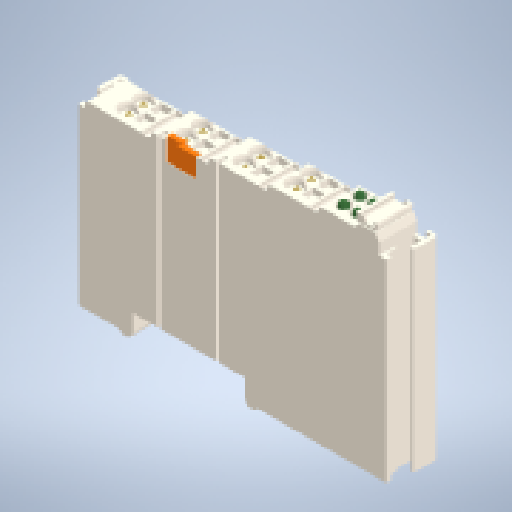
# Autodesk Inventor part: 750-408
Saved by Autodesk Inventor 2025.3 (Build 293356000, 356)
## iProperties
Category: PARTsolutions
Company: WAGO
Created: 2026-07-30
Part Number: 750-408
Material: Generic
Catalog Web Link: www.3dfindit.com
Description: 750-408-4-CHANNEL DIGITAL INPUT MODULE DC 24 V 3,0 ms
Vendor: WAGO
Document SubType Name: Modeling
Designer: psAdmin
Manufacturer: WAGO
Mass: 46.5 g
Surface Area: 195.349 cm^2
Volume: 66.2406 cm^3
Density: 1 g/cm^3
Appearance: PSOLRGB-222-214-201
Categories: <MemberInstance><Categories><Category DisplayName="" Mnemonic="CABLEANDHARNESS" InternalName="e4a7e005-5e42-4d16-b293-125e7f0d0512"><Category DisplayName="" Mnemonic="CONNECTORS" InternalName="6f634eba-a678-4820-a31d-2c2d5ee6728e"><CategoryParameter DisplayName="" Mnemonic="REFDES" InternalName="c3740e8c-60ab-4d5d-8584-52b73222f2f0"/><Category DisplayName="" Mnemonic="DISCRETEWIRE" InternalName="9a3407de-09b2-4cdb-8c40-9708d5144a28"/></Category></Category></Categories><FamilyTemplate><FamilyTemplateParameters></FamilyTemplateParameters></FamilyTemplate><CategoryParameterMap><ParamToTemplateMap><ParamToTemplate CategoryParameter="//CategoryParameter[@InternalName='c3740e8c-60ab-4d5d-8584-52b73222f2f0']" ConstantValue=""/></ParamToTemplateMap></CategoryParameterMap></MemberInstance>
PSOL_IDENT_0: {$CADENAS_DATA/23d-libs/wago/pg15/serie750/0750-0408_0999-0962.prj},156 {VTYP=3D},{NB=750-408},{LINA=
PSOL_IDENT_1: 750-408},{NN=750-408},{DATE=29.04.2026 11:59:08},{GEOMDATE=18.07.2023 08:27:45},{VERSION=},{LINEID=6
PSOL_IDENT_2: 40},{WBVAR=},{WBNUMERIC=}  {NB=750-408},{LINA=750-408},{KT=DUMMY},{BESTNR=750-408},{INFODE=Info DE},
PSOL_IDENT_3: {INFOEN=Info EN},{QUERSCHNITT1=0.08 - 2.5},{QUERSCHNITT2=28 - 14},{ABISOLIERLAENGE=8 - 9},{HOEHE=64.
PSOL_IDENT_4: 00},{BREITE=12.00},{TIEFE=100.00},{FARBE=lichtgrau},{GEWICHT=46.500},{BEMERKUNGEN=24V DC 3.0 ms  |
PSOL_IDENT_5: negativ schaltend},{RGB=0.87,0.84,0.79,0},{ECLASS71=27-24-26-04},{LINKDE=http://www.wago.com/de/p/75
PSOL_IDENT_6: 0-408},{LINKEN=http://www.wago.com/global/p/750-408},{FILENAME=750-408}
NB: 750-408
NN: 750-408
NT: 4-CHANNEL DIGITAL INPUT MODULE DC 24 V 3,0 ms
NBSYN: $BESTNR.
LINA: 750-408
CATALOG: WAGO
OFFICIAL_STANDARD_NUMBERS: NO
BESTNR: 750-408
INFODE: Info DE
INFOEN: Info EN
QUERSCHNITT1: 0.08 - 2.5
QUERSCHNITT2: 28 - 14
ABISOLIERLAENGE: 8 - 9
HOEHE: 64
BREITE: 12
TIEFE: 100
FARBE: lichtgrau
GEWICHT: 46.5
BEMERKUNGEN: 24V DC 3.0 ms  |  negativ schaltend
ECLASS71: 27-24-26-04
SUPPLIER: WAGO
ARTICLENO: 750-408
BOMINFO: 750-408
CREATOR: CADENAS GmbH
Title: 750-408
Author: Cadenas PARTsolutions
Comments: 4-CHANNEL DIGITAL INPUT MODULE DC 24 V 3,0 ms
Autodesk Inventor part; units mm, degrees
sketch "Skizze_1" plane through (0, 0, 0) normal (0, 0, 1) x (1, 0, 0)
  line L0 (-32.4, 49.7072) -> (-32.4, -6.4)
  line L1 (-32.4, -6.4) -> (-21.9679, -6.4)
  line L2 (-21.9679, -6.4) -> (-20.7, -7.1321)
  arc A0 (-20.7, -7.1321) -> (-17.7, -5.4) centre (-19.7, -5.4) ccw
  line L3 (-17.7, -5.4) -> (-17.7, 0)
  line L4 (-17.7, 0) -> (17.7, 0)
  line L5 (17.7, 0) -> (17.7, -5.4)
  arc A1 (17.7, -5.4) -> (20.7, -7.1321) centre (19.7, -5.4) ccw
  line L6 (20.7, -7.1321) -> (21.9679, -6.4)
  line L7 (21.9679, -6.4) -> (60, -6.4)
  line L8 (60, -6.4) -> (60, 57.9215)
  line L9 (60, 57.9215) -> (58.8, 60)
  line L10 (58.8, 60) -> (54.2, 60)
  arc A2 (54.2, 60) -> (53.5405, 59.7517) centre (54.2, 59) ccw
  line L11 (53.5405, 59.7517) -> (52, 58.4)
  line L12 (52, 58.4) -> (41.9117, 58.4)
  line L13 (41.9117, 58.4) -> (41.8025, 58.3537)
  line L14 (41.8025, 58.3537) -> (41.6531, 58.1989)
  arc A3 (41.6531, 58.1989) -> (41.8439, 57.6405) centre (41.8915, 57.9686) ccw
  arc A4 (42.2357, 56.9584) -> (41.8439, 57.6405) centre (41.7721, 57.1457) ccw
  line L15 (42.2357, 56.9584) -> (42.1581, 56.7664)
  line L16 (42.1581, 56.7664) -> (38.0948, 55.0416)
  line L17 (38.0948, 55.0416) -> (37.9028, 55.1192)
  arc A5 (37.6842, 55.8749) -> (37.9028, 55.1192) centre (38.0901, 55.5828) ccw
  arc A6 (37.6842, 55.8749) -> (37.4152, 56.4) centre (37.4152, 56.0685) ccw
  line L18 (37.4152, 56.4) -> (25.9117, 56.4)
  line L19 (25.9117, 56.4) -> (25.8025, 56.3537)
  line L20 (25.8025, 56.3537) -> (25.6531, 56.1989)
  arc A7 (25.6531, 56.1989) -> (25.8439, 55.6405) centre (25.8915, 55.9686) ccw
  arc A8 (26.2357, 54.9584) -> (25.8439, 55.6405) centre (25.7721, 55.1457) ccw
  line L21 (26.2357, 54.9584) -> (26.1581, 54.7664)
  line L22 (26.1581, 54.7664) -> (22.0948, 53.0416)
  line L23 (22.0948, 53.0416) -> (21.9028, 53.1192)
  arc A9 (21.6842, 53.8749) -> (21.9028, 53.1192) centre (22.0901, 53.5828) ccw
  arc A10 (21.6842, 53.8749) -> (21.4152, 54.4) centre (21.4152, 54.0685) ccw
  line L24 (21.4152, 54.4) -> (7.5117, 54.4)
  line L25 (7.5117, 54.4) -> (7.4025, 54.3537)
  line L26 (7.4025, 54.3537) -> (7.2531, 54.1989)
  arc A11 (7.2531, 54.1989) -> (7.4439, 53.6405) centre (7.4915, 53.9686) ccw
  arc A12 (7.8357, 52.9584) -> (7.4439, 53.6405) centre (7.3721, 53.1457) ccw
  line L27 (7.8357, 52.9584) -> (7.7581, 52.7664)
  line L28 (7.7581, 52.7664) -> (3.6948, 51.0416)
  line L29 (3.6948, 51.0416) -> (3.5028, 51.1192)
  arc A13 (3.2842, 51.8749) -> (3.5028, 51.1192) centre (3.6901, 51.5828) ccw
  arc A14 (3.2842, 51.8749) -> (3.0152, 52.4) centre (3.0152, 52.0685) ccw
  line L30 (3.0152, 52.4) -> (-10.8883, 52.4)
  line L31 (-10.8883, 52.4) -> (-10.9975, 52.3537)
  line L32 (-10.9975, 52.3537) -> (-11.1469, 52.1989)
  arc A15 (-11.1469, 52.1989) -> (-10.9561, 51.6405) centre (-10.9085, 51.9686) ccw
  arc A16 (-10.5643, 50.9584) -> (-10.9561, 51.6405) centre (-11.0279, 51.1457) ccw
  line L33 (-10.5643, 50.9584) -> (-10.6419, 50.7664)
  line L34 (-10.6419, 50.7664) -> (-14.7052, 49.0416)
  line L35 (-14.7052, 49.0416) -> (-14.8972, 49.1192)
  arc A17 (-15.1158, 49.8749) -> (-14.8972, 49.1192) centre (-14.7099, 49.5828) ccw
  arc A18 (-15.1158, 49.8749) -> (-15.3848, 50.4) centre (-15.3848, 50.0685) ccw
  line L36 (-15.3848, 50.4) -> (-32, 50.4)
  line L37 (-32, 50.4) -> (-32.4, 49.7072)
  constraints: 76 end point, 38 point on circle, 19 centre point
extrude "Extrusion1" add sketch "Skizze_1" along normal blind 12
sketch "Skizze_10" plane through (0, 0, 0) normal (0, 0, 1) x (1, 0, 0)
  line L0 (37.2, 56.4) -> (37.9815, 54.559)
  line L1 (37.9815, 54.559) -> (42.6932, 56.559)
  line L2 (42.6932, 56.559) -> (41.9117, 58.4)
  line L3 (41.9117, 58.4) -> (41.3423, 58.1583)
  arc A0 (41.3423, 58.1583) -> (40.8125, 56.8471) centre (41.733, 57.2378) ccw
  line L4 (40.8125, 56.8471) -> (38.9715, 56.0656)
  arc A1 (38.9715, 56.0656) -> (37.6603, 56.5954) centre (38.051, 55.6749) ccw
  line L5 (37.6603, 56.5954) -> (37.2, 56.4)
  constraints: 12 end point, 4 point on circle, 2 centre point
extrude "Extrusion2" add sketch "Skizze_10" along normal blind 0.5
sketch "Skizze_11" plane through (0, 0, 0) normal (0, 0, 1) x (1, 0, 0)
  line L0 (21.2, 54.4) -> (21.9815, 52.559)
  line L1 (21.9815, 52.559) -> (26.6932, 54.559)
  line L2 (26.6932, 54.559) -> (25.9117, 56.4)
  line L3 (25.9117, 56.4) -> (25.3423, 56.1583)
  arc A0 (25.3423, 56.1583) -> (24.8125, 54.8471) centre (25.733, 55.2378) ccw
  line L4 (24.8125, 54.8471) -> (22.9715, 54.0656)
  arc A1 (22.9715, 54.0656) -> (21.6603, 54.5954) centre (22.051, 53.6749) ccw
  line L5 (21.6603, 54.5954) -> (21.2, 54.4)
  constraints: 12 end point, 4 point on circle, 2 centre point
extrude "Extrusion3" add sketch "Skizze_11" along normal blind 0.5
sketch "Skizze_12" plane through (0, 0, 0) normal (0, 0, 1) x (1, 0, 0)
  line L0 (2.8, 52.4) -> (3.5815, 50.559)
  line L1 (3.5815, 50.559) -> (8.2932, 52.559)
  line L2 (8.2932, 52.559) -> (7.5117, 54.4)
  line L3 (7.5117, 54.4) -> (6.9423, 54.1583)
  arc A0 (6.9423, 54.1583) -> (6.4125, 52.8471) centre (7.333, 53.2378) ccw
  line L4 (6.4125, 52.8471) -> (4.5715, 52.0656)
  arc A1 (4.5715, 52.0656) -> (3.2603, 52.5954) centre (3.651, 51.6749) ccw
  line L5 (3.2603, 52.5954) -> (2.8, 52.4)
  constraints: 12 end point, 4 point on circle, 2 centre point
extrude "Extrusion4" add sketch "Skizze_12" along normal blind 0.5
sketch "Skizze_13" plane through (0, 0, 0) normal (0, 0, 1) x (1, 0, 0)
  line L0 (-15.6, 50.4) -> (-14.8185, 48.559)
  line L1 (-14.8185, 48.559) -> (-10.1068, 50.559)
  line L2 (-10.1068, 50.559) -> (-10.8883, 52.4)
  line L3 (-10.8883, 52.4) -> (-11.4577, 52.1583)
  arc A0 (-11.4577, 52.1583) -> (-11.9875, 50.8471) centre (-11.067, 51.2378) ccw
  line L4 (-11.9875, 50.8471) -> (-13.8285, 50.0656)
  arc A1 (-13.8285, 50.0656) -> (-15.1397, 50.5954) centre (-14.749, 49.6749) ccw
  line L5 (-15.1397, 50.5954) -> (-15.6, 50.4)
  constraints: 12 end point, 4 point on circle, 2 centre point
extrude "Extrusion5" add sketch "Skizze_13" along normal blind 0.5
sketch "Skizze_14" plane through (0, 0, 12) normal (0, 0, 1) x (1, 0, 0)
  line L0 (37.2, 56.4) -> (37.9815, 54.559)
  line L1 (37.9815, 54.559) -> (42.6932, 56.559)
  line L2 (42.6932, 56.559) -> (41.9117, 58.4)
  line L3 (41.9117, 58.4) -> (41.3423, 58.1583)
  arc A0 (41.3423, 58.1583) -> (40.8125, 56.8471) centre (41.733, 57.2378) ccw
  line L4 (40.8125, 56.8471) -> (38.9715, 56.0656)
  arc A1 (38.9715, 56.0656) -> (37.6603, 56.5954) centre (38.051, 55.6749) ccw
  line L5 (37.6603, 56.5954) -> (37.2, 56.4)
  constraints: 12 end point, 4 point on circle, 2 centre point
extrude "Extrusion6" add sketch "Skizze_14" against normal blind 0.5
sketch "Skizze_15" plane through (0, 0, 12) normal (0, 0, 1) x (1, 0, 0)
  line L0 (21.2, 54.4) -> (21.9815, 52.559)
  line L1 (21.9815, 52.559) -> (26.6932, 54.559)
  line L2 (26.6932, 54.559) -> (25.9117, 56.4)
  line L3 (25.9117, 56.4) -> (25.3423, 56.1583)
  arc A0 (25.3423, 56.1583) -> (24.8125, 54.8471) centre (25.733, 55.2378) ccw
  line L4 (24.8125, 54.8471) -> (22.9715, 54.0656)
  arc A1 (22.9715, 54.0656) -> (21.6603, 54.5954) centre (22.051, 53.6749) ccw
  line L5 (21.6603, 54.5954) -> (21.2, 54.4)
  constraints: 12 end point, 4 point on circle, 2 centre point
extrude "Extrusion7" add sketch "Skizze_15" against normal blind 0.5
sketch "Skizze_16" plane through (0, 0, 12) normal (0, 0, 1) x (1, 0, 0)
  line L0 (2.8, 52.4) -> (3.5815, 50.559)
  line L1 (3.5815, 50.559) -> (8.2932, 52.559)
  line L2 (8.2932, 52.559) -> (7.5117, 54.4)
  line L3 (7.5117, 54.4) -> (6.9423, 54.1583)
  arc A0 (6.9423, 54.1583) -> (6.4125, 52.8471) centre (7.333, 53.2378) ccw
  line L4 (6.4125, 52.8471) -> (4.5715, 52.0656)
  arc A1 (4.5715, 52.0656) -> (3.2603, 52.5954) centre (3.651, 51.6749) ccw
  line L5 (3.2603, 52.5954) -> (2.8, 52.4)
  constraints: 12 end point, 4 point on circle, 2 centre point
extrude "Extrusion8" add sketch "Skizze_16" against normal blind 0.5
sketch "Skizze_17" plane through (0, 0, 12) normal (0, 0, 1) x (1, 0, 0)
  line L0 (-15.6, 50.4) -> (-14.8185, 48.559)
  line L1 (-14.8185, 48.559) -> (-10.1068, 50.559)
  line L2 (-10.1068, 50.559) -> (-10.8883, 52.4)
  line L3 (-10.8883, 52.4) -> (-11.4577, 52.1583)
  arc A0 (-11.4577, 52.1583) -> (-11.9875, 50.8471) centre (-11.067, 51.2378) ccw
  line L4 (-11.9875, 50.8471) -> (-13.8285, 50.0656)
  arc A1 (-13.8285, 50.0656) -> (-15.1397, 50.5954) centre (-14.749, 49.6749) ccw
  line L5 (-15.1397, 50.5954) -> (-15.6, 50.4)
  constraints: 12 end point, 4 point on circle, 2 centre point
extrude "Extrusion9" add sketch "Skizze_17" against normal blind 0.5
sketch "Skizze_46" plane through (0, 0, 12) normal (0, 0, 1) x (1, 0, 0)
  line L0 (-7.3, 46.4) -> (2.5, 46.4)
  line L1 (2.5, 46.4) -> (2.5, 52.4)
  line L2 (2.5, 52.4) -> (-7.3, 52.4)
  line L3 (-7.3, 52.4) -> (-7.3, 46.4)
  constraints: 8 end point
extrude "Extrusion10" cut sketch "Skizze_46" against normal blind 1.9
sketch "Skizze_47" plane through (0, 0, 11.05) normal (0, 0, 1) x (1, 0, 0)
  line L0 (-7, 53.4) -> (-7, 46.6)
  arc A0 (-7, 46.6) -> (-6.8, 46.4) centre (-6.8, 46.6) ccw
  line L1 (-6.8, 46.4) -> (2, 46.4)
  arc A1 (2, 46.4) -> (2.2, 46.6) centre (2, 46.6) ccw
  line L2 (2.2, 46.6) -> (2.2, 52.2)
  arc A2 (2.2, 52.2) -> (2, 52.4) centre (2, 52.2) ccw
  line L3 (2, 52.4) -> (-3.3, 52.4)
  arc A3 (-3.3305, 52.9984) -> (-3.3, 52.4) centre (-3.3, 52.7) ccw
  line L4 (-3.3305, 52.9984) -> (-2.3246, 53.1013)
  arc A4 (-2.3246, 53.1013) -> (-2.35, 53.6) centre (-2.35, 53.35) ccw
  line L5 (-2.35, 53.6) -> (-6.8, 53.6)
  arc A5 (-6.8, 53.6) -> (-7, 53.4) centre (-6.8, 53.4) ccw
  constraints: 12 end point, 12 point on circle, 6 centre point
extrude "Extrusion11" add sketch "Skizze_47" along normal mid plane 1.6
sketch "Skizze_2" plane through (0, -6.4, 0) normal (0, 1, 0) x (1, 0, 0)
  line L0 (60, 0) -> (60, -1.7)
  arc A0 (60.5, -1.2) -> (60, -1.7) centre (60.5, -1.7) ccw
  line L1 (60.5, -1.2) -> (61.9, -1.2)
  arc A1 (62.4, -1.7) -> (61.9, -1.2) centre (61.9, -1.7) ccw
  line L2 (62.4, -1.7) -> (62.4, -4.3)
  arc A2 (62.4, -4.3) -> (63.8, -4.3) centre (63.1, -4.3) ccw
  line L3 (63.8, -4.3) -> (63.8, 1.8)
  arc A3 (63.8, 1.8) -> (62.8, 2.8) centre (62.8, 1.8) ccw
  line L4 (62.8, 2.8) -> (61.3, 2.8)
  arc A4 (61.3, 2.8) -> (60.8, 2.3) centre (61.3, 2.3) ccw
  line L5 (60.8, 2.3) -> (60.8, 1.9)
  arc A5 (60.8, 1.9) -> (61, 1.7) centre (61, 1.9) ccw
  line L6 (61, 1.7) -> (62.2, 1.7)
  arc A6 (62.4, 1.5) -> (62.2, 1.7) centre (62.2, 1.5) ccw
  line L7 (62.4, 1.5) -> (62.4, 0.2)
  arc A7 (62.2, 0) -> (62.4, 0.2) centre (62.2, 0.2) ccw
  line L8 (62.2, 0) -> (60, 0)
  constraints: 18 end point, 16 point on circle, 8 centre point
extrude "Extrusion12" add sketch "Skizze_2" along normal blind 60.8
sketch "Skizze_3" plane through (0, -6.4, 0) normal (0, 1, 0) x (1, 0, 0)
  arc A0 (-36.2, -4.3) -> (-34.8, -4.3) centre (-35.5, -4.3) ccw
  line L0 (-34.8, -4.3) -> (-34.8, -1.7)
  arc A1 (-34.3, -1.2) -> (-34.8, -1.7) centre (-34.3, -1.7) ccw
  line L1 (-34.3, -1.2) -> (-32.9, -1.2)
  arc A2 (-32.4, -1.7) -> (-32.9, -1.2) centre (-32.9, -1.7) ccw
  line L2 (-32.4, -1.7) -> (-32.4, 0)
  line L3 (-32.4, 0) -> (-34.6, 0)
  arc A3 (-34.8, 0.2) -> (-34.6, 0) centre (-34.6, 0.2) ccw
  line L4 (-34.8, 0.2) -> (-34.8, 1.5)
  arc A4 (-34.6, 1.7) -> (-34.8, 1.5) centre (-34.6, 1.5) ccw
  line L5 (-34.6, 1.7) -> (-33.4, 1.7)
  arc A5 (-33.4, 1.7) -> (-33.2, 1.9) centre (-33.4, 1.9) ccw
  line L6 (-33.2, 1.9) -> (-33.2, 2.3)
  arc A6 (-33.2, 2.3) -> (-33.7, 2.8) centre (-33.7, 2.3) ccw
  line L7 (-33.7, 2.8) -> (-35.2, 2.8)
  arc A7 (-35.2, 2.8) -> (-36.2, 1.8) centre (-35.2, 1.8) ccw
  line L8 (-36.2, 1.8) -> (-36.2, -4.3)
  constraints: 18 end point, 16 point on circle, 8 centre point
extrude "Extrusion13" add sketch "Skizze_3" along normal blind 54.8
sketch "Skizze_9" plane through (0, -6.4, 0) normal (0, 1, 0) x (1, 0, 0)
  line L0 (-34.6, -10.6) -> (-34.6, -11.8)
  arc A0 (-34.6, -11.8) -> (-34.4, -12) centre (-34.4, -11.8) ccw
  line L1 (-34.4, -12) -> (-32.4, -12)
  line L2 (-32.4, -12) -> (-32.4, -7)
  line L3 (-32.4, -7) -> (-33, -7)
  line L4 (-33, -7) -> (-33, -10.4)
  line L5 (-33, -10.4) -> (-34.4, -10.4)
  arc A1 (-34.4, -10.4) -> (-34.6, -10.6) centre (-34.4, -10.6) ccw
  constraints: 12 end point, 4 point on circle, 2 centre point
extrude "Extrusion14" add sketch "Skizze_9" along normal blind 54.8
sketch "Skizze_8" plane through (0, -6.4, 0) normal (0, 1, 0) x (1, 0, 0)
  line L0 (60, -7) -> (60, -12)
  line L1 (60, -12) -> (62, -12)
  arc A0 (62, -12) -> (62.2, -11.8) centre (62, -11.8) ccw
  line L2 (62.2, -11.8) -> (62.2, -10.6)
  arc A1 (62.2, -10.6) -> (62, -10.4) centre (62, -10.6) ccw
  line L3 (62, -10.4) -> (60.6, -10.4)
  line L4 (60.6, -10.4) -> (60.6, -7)
  line L5 (60.6, -7) -> (60, -7)
  constraints: 12 end point, 4 point on circle, 2 centre point
extrude "Extrusion15" add sketch "Skizze_8" along normal blind 60.8
sketch "Skizze_4" plane through (49, 0, 0) normal (1, 0, 0) x (0, 0, -1)
  line L0 (-2.7, 56.4) -> (-2.7, 58.4)
  line L1 (-2.7, 58.4) -> (-0.6, 58.4)
  line L2 (-0.6, 58.4) -> (-0.6, 58)
  line L3 (-0.6, 58) -> (-1, 57.6)
  line L4 (-1, 57.6) -> (-1, 56.4)
  line L5 (-1, 56.4) -> (-2.7, 56.4)
  line L6 (-2.7, 56.4) -> (-2.7, 58.4)
  constraints: 14 end point
revolve "Revolution1" cut sketch "Skizze_4" angle 360 about axis through (49, 56.4, 2.7) along (0, -1, 0)
pattern_linear "Rectangular Pattern1" count 2 spacing 5 along (0, 0, 1) of "Revolution1"
sketch "Skizze_6" plane through (49, 0, 0) normal (1, 0, 0) x (0, 0, -1)
  line L0 (-2.7, 55.4) -> (-2.7, 59.7)
  arc A0 (-1.25, 58.25) -> (-2.7, 59.7) centre (-2.7, 58.25) ccw
  line L1 (-1.25, 58.25) -> (-1.25, 56.42)
  line L2 (-1.25, 56.42) -> (-1.15, 56.42)
  line L3 (-1.15, 56.42) -> (-1.15, 55.4)
  line L4 (-1.15, 55.4) -> (-2.7, 55.4)
  line L5 (-2.7, 55.4) -> (-2.7, 59.7)
  constraints: 12 end point, 2 point on circle, 1 centre point
revolve "Revolution2" add sketch "Skizze_6" angle 360 about axis through (49, 55.4, 2.7) along (0, -1, 0)
pattern_linear "Rectangular Pattern2" count 2 spacing 5 along (0, 0, 1) of "Revolution2"
sketch "Skizze_18" plane through (44.6, 0, 0) normal (1, 0, 0) x (0, 0, -1)
  line L0 (-2.7, 56.4) -> (-2.7, 58.4)
  line L1 (-2.7, 58.4) -> (-0.6, 58.4)
  line L2 (-0.6, 58.4) -> (-0.6, 58)
  line L3 (-0.6, 58) -> (-1, 57.6)
  line L4 (-1, 57.6) -> (-1, 56.4)
  line L5 (-1, 56.4) -> (-2.7, 56.4)
  line L6 (-2.7, 56.4) -> (-2.7, 58.4)
  constraints: 14 end point
revolve "Revolution3" cut sketch "Skizze_18" angle 360 about axis through (44.6, 56.4, 2.7) along (0, -1, 0)
pattern_linear "Rectangular Pattern3" count 2 spacing 5 along (0, 0, 1) of "Revolution3"
sketch "Skizze_20" plane through (44.6, 0, 0) normal (1, 0, 0) x (0, 0, -1)
  line L0 (-2.7, 55.4) -> (-2.7, 59.7)
  arc A0 (-1.25, 58.25) -> (-2.7, 59.7) centre (-2.7, 58.25) ccw
  line L1 (-1.25, 58.25) -> (-1.25, 56.42)
  line L2 (-1.25, 56.42) -> (-1.15, 56.42)
  line L3 (-1.15, 56.42) -> (-1.15, 55.4)
  line L4 (-1.15, 55.4) -> (-2.7, 55.4)
  line L5 (-2.7, 55.4) -> (-2.7, 59.7)
  constraints: 12 end point, 2 point on circle, 1 centre point
revolve "Revolution4" add sketch "Skizze_20" angle 360 about axis through (44.6, 55.4, 2.7) along (0, -1, 0)
pattern_linear "Rectangular Pattern4" count 2 spacing 5 along (0, 0, 1) of "Revolution4"
sketch "Sketch20" plane through (25.9117, 56.4, 12) normal (0, 1, 0) x (1, 0, 0)
  point P0 (3.1883, 9.5)
hole "Hole1" at (29.1, 56.4, 2.5) direction (0, -1, 0) diameter 4.2 depth 2 countersink diameter 5.4 countersink angle 90
pattern_linear "Rectangular Pattern5" count 2 spacing 5 along (0, 0, 1) of "Hole1"
sketch "Skizze_24" plane through (31.2, 0, 0) normal (1, 0, 0) x (0, 0, -1)
  line L0 (-2.5, 54.4) -> (-2.5, 56.4)
  line L1 (-2.5, 56.4) -> (-1.2, 56.4)
  line L2 (-1.2, 56.4) -> (-1.4, 55.8)
  line L3 (-1.4, 55.8) -> (-1.4, 54.4)
  line L4 (-1.4, 54.4) -> (-2.5, 54.4)
  line L5 (-2.5, 54.4) -> (-2.5, 56.4)
  constraints: 12 end point
revolve "Revolution5" cut sketch "Skizze_24" angle 360 about axis through (31.2, 54.4, 2.5) along (0, -1, 0)
pattern_linear "Rectangular Pattern6" count 2 spacing 5 along (0, 0, 1) of "Revolution5"
sketch "Skizze_26" plane through (33, 0, 0) normal (1, 0, 0) x (0, 0, -1)
  line L0 (-4.5, 54.4) -> (-0.8, 54.4)
  line L1 (-0.8, 54.4) -> (-0.8, 56.4)
  line L2 (-0.8, 56.4) -> (-4.5, 56.4)
  line L3 (-4.5, 56.4) -> (-4.5, 54.4)
  constraints: 8 end point
extrude "Extrusion16" cut sketch "Skizze_26" along normal blind 3.8
pattern_linear "Rectangular Pattern7" count 2 spacing 5 along (0, 0, 1) of "Extrusion16"
sketch "Sketch23" plane through (7.5117, 54.4, 12) normal (0, 1, 0) x (1, 0, 0)
  point P0 (5.5883, 9.5)
hole "Hole2" at (13.1, 54.4, 2.5) direction (0, -1, 0) diameter 4.2 depth 2 countersink diameter 5.4 countersink angle 90
pattern_linear "Rectangular Pattern8" count 2 spacing 5 along (0, 0, 1) of "Hole2"
sketch "Skizze_30" plane through (15.2, 0, 0) normal (1, 0, 0) x (0, 0, -1)
  line L0 (-2.5, 52.4) -> (-2.5, 54.4)
  line L1 (-2.5, 54.4) -> (-1.2, 54.4)
  line L2 (-1.2, 54.4) -> (-1.4, 53.8)
  line L3 (-1.4, 53.8) -> (-1.4, 52.4)
  line L4 (-1.4, 52.4) -> (-2.5, 52.4)
  line L5 (-2.5, 52.4) -> (-2.5, 54.4)
  constraints: 12 end point
revolve "Revolution6" cut sketch "Skizze_30" angle 360 about axis through (15.2, 52.4, 2.5) along (0, -1, 0)
pattern_linear "Rectangular Pattern9" count 2 spacing 5 along (0, 0, 1) of "Revolution6"
sketch "Skizze_32" plane through (17, 0, 0) normal (1, 0, 0) x (0, 0, -1)
  line L0 (-4.5, 52.4) -> (-0.8, 52.4)
  line L1 (-0.8, 52.4) -> (-0.8, 54.4)
  line L2 (-0.8, 54.4) -> (-4.5, 54.4)
  line L3 (-4.5, 54.4) -> (-4.5, 52.4)
  constraints: 8 end point
extrude "Extrusion17" cut sketch "Skizze_32" along normal blind 3.8
pattern_linear "Rectangular Pattern10" count 2 spacing 5 along (0, 0, 1) of "Extrusion17"
sketch "Sketch26" plane through (-10.8883, 52.4, 12) normal (0, 1, 0) x (1, 0, 0)
  point P0 (5.5883, 9.5)
hole "Hole3" at (-5.3, 52.4, 2.5) direction (0, -1, 0) diameter 4.2 depth 2 countersink diameter 5.4 countersink angle 90
pattern_linear "Rectangular Pattern11" count 2 spacing 5 along (0, 0, 1) of "Hole3"
sketch "Skizze_36" plane through (-3.2, 0, 0) normal (1, 0, 0) x (0, 0, -1)
  line L0 (-2.5, 50.4) -> (-2.5, 52.4)
  line L1 (-2.5, 52.4) -> (-1.2, 52.4)
  line L2 (-1.2, 52.4) -> (-1.4, 51.8)
  line L3 (-1.4, 51.8) -> (-1.4, 50.4)
  line L4 (-1.4, 50.4) -> (-2.5, 50.4)
  line L5 (-2.5, 50.4) -> (-2.5, 52.4)
  constraints: 12 end point
revolve "Revolution7" cut sketch "Skizze_36" angle 360 about axis through (-3.2, 50.4, 2.5) along (0, -1, 0)
pattern_linear "Rectangular Pattern12" count 2 spacing 5 along (0, 0, 1) of "Revolution7"
sketch "Skizze_38" plane through (-1.4, 0, 0) normal (1, 0, 0) x (0, 0, -1)
  line L0 (-4.5, 50.4) -> (-0.8, 50.4)
  line L1 (-0.8, 50.4) -> (-0.8, 52.4)
  line L2 (-0.8, 52.4) -> (-4.5, 52.4)
  line L3 (-4.5, 52.4) -> (-4.5, 50.4)
  constraints: 8 end point
extrude "Extrusion18" cut sketch "Skizze_38" along normal blind 3.8
pattern_linear "Rectangular Pattern13" count 2 spacing 5 along (0, 0, 1) of "Extrusion18"
sketch "Sketch29" plane through (-32, 50.4, 12) normal (0, 1, 0) x (1, 0, 0)
  point P0 (8.3, 9.5)
hole "Hole4" at (-23.7, 50.4, 2.5) direction (0, -1, 0) diameter 4.2 depth 2 countersink diameter 5.4 countersink angle 90
pattern_linear "Rectangular Pattern14" count 2 spacing 5 along (0, 0, 1) of "Hole4"
sketch "Skizze_42" plane through (-21.6, 0, 0) normal (1, 0, 0) x (0, 0, -1)
  line L0 (-2.5, 48.4) -> (-2.5, 50.4)
  line L1 (-2.5, 50.4) -> (-1.2, 50.4)
  line L2 (-1.2, 50.4) -> (-1.4, 49.8)
  line L3 (-1.4, 49.8) -> (-1.4, 48.4)
  line L4 (-1.4, 48.4) -> (-2.5, 48.4)
  line L5 (-2.5, 48.4) -> (-2.5, 50.4)
  constraints: 12 end point
revolve "Revolution8" cut sketch "Skizze_42" angle 360 about axis through (-21.6, 48.4, 2.5) along (0, -1, 0)
pattern_linear "Rectangular Pattern15" count 2 spacing 5 along (0, 0, 1) of "Revolution8"
sketch "Skizze_44" plane through (-19.8, 0, 0) normal (1, 0, 0) x (0, 0, -1)
  line L0 (-4.5, 48.4) -> (-0.8, 48.4)
  line L1 (-0.8, 48.4) -> (-0.8, 50.4)
  line L2 (-0.8, 50.4) -> (-4.5, 50.4)
  line L3 (-4.5, 50.4) -> (-4.5, 48.4)
  constraints: 8 end point
extrude "Extrusion19" cut sketch "Skizze_44" along normal blind 3.8
pattern_linear "Rectangular Pattern16" count 2 spacing 5 along (0, 0, 1) of "Extrusion19"
sketch "Skizze_48" plane through (0, 0, 6) normal (0, 0, 1) x (1, 0, 0)
  line L0 (52.1, 61.9) -> (52.5, 61.9)
  line L1 (52.5, 61.9) -> (52.5, 60.5)
  arc A0 (52.5, 60.5) -> (53, 60) centre (53, 60.5) ccw
  line L2 (53, 60) -> (58.4, 60)
  arc A1 (58.4, 60) -> (58.9, 60.5) centre (58.4, 60.5) ccw
  line L3 (58.9, 60.5) -> (58.9, 61.9)
  line L4 (58.9, 61.9) -> (59.3, 61.9)
  arc A2 (59.3, 61.9) -> (58.8, 62.4) centre (58.8, 61.9) ccw
  line L5 (58.8, 62.4) -> (58.1, 62.4)
  arc A3 (58.1, 62.4) -> (57.86, 61.92) centre (58.1, 62.1) ccw
  line L6 (57.86, 61.92) -> (58.1, 61.6)
  arc A4 (57.7, 60.8) -> (58.1, 61.6) centre (57.7, 61.3) ccw
  line L7 (57.7, 60.8) -> (53.7, 60.8)
  arc A5 (53.3, 61.6) -> (53.7, 60.8) centre (53.7, 61.3) ccw
  line L8 (53.3, 61.6) -> (53.54, 61.92)
  arc A6 (53.54, 61.92) -> (53.3, 62.4) centre (53.3, 62.1) ccw
  line L9 (53.3, 62.4) -> (52.6, 62.4)
  arc A7 (52.6, 62.4) -> (52.1, 61.9) centre (52.6, 61.9) ccw
  constraints: 20 end point, 16 point on circle, 8 centre point
extrude "Extrusion20" add sketch "Skizze_48" along normal mid plane 11.2
sketch "Skizze_49" plane through (0, 0, 11.6) normal (0, 0, 1) x (1, 0, 0)
  line L0 (53.2, 62.4) -> (53.2, 60.8)
  line L1 (53.2, 60.8) -> (55.1, 60.8)
  line L2 (55.1, 60.8) -> (54.8699, 61.6588)
  arc A0 (54.8699, 61.6588) -> (53.904, 62.4) centre (53.904, 61.4) ccw
  line L3 (53.904, 62.4) -> (53.2, 62.4)
  constraints: 8 end point, 2 point on circle, 1 centre point
extrude "Extrusion21" add sketch "Skizze_49" against normal blind 0.6
sketch "Skizze_50" plane through (0, 0, 0.4) normal (0, 0, 1) x (1, 0, 0)
  line L0 (56.3, 60.8) -> (58.2, 60.8)
  line L1 (58.2, 60.8) -> (58.2, 62.4)
  line L2 (58.2, 62.4) -> (57.496, 62.4)
  arc A0 (57.496, 62.4) -> (56.5301, 61.6588) centre (57.496, 61.4) ccw
  line L3 (56.5301, 61.6588) -> (56.3, 60.8)
  constraints: 8 end point, 2 point on circle, 1 centre point
extrude "Extrusion22" add sketch "Skizze_50" along normal blind 0.6
sketch "Sketch_1" plane through (0, -10, 0) normal (0, 1, 0) x (1, 0, 0)
  line L0 (-9.7, -13) -> (9.7, -13)
  line L1 (9.7, -13) -> (9.7, -9.4)
  line L2 (9.7, -9.4) -> (8.7, -9.4)
  line L3 (8.7, -9.4) -> (8.7, -12)
  line L4 (8.7, -12) -> (-8.7, -12)
  line L5 (-8.7, -12) -> (-8.7, -9.4)
  line L6 (-8.7, -9.4) -> (-9.7, -9.4)
  line L7 (-9.7, -9.4) -> (-9.7, -13)
  constraints: 16 end point
extrude "Extrusion23" cut sketch "Sketch_1" along normal blind 65
sketch "Sketch_2" plane through (0, 0, 0) normal (0, 0, 1) x (1, 0, 0)
  line L0 (8.95, 44.9) -> (8.95, 41.3)
  line L1 (8.95, 41.3) -> (9.35, 41.3)
  line L2 (9.35, 41.3) -> (9.35, 44.9)
  line L3 (9.35, 44.9) -> (8.95, 44.9)
  constraints: 8 end point
extrude "Extrusion24" add sketch "Sketch_2" against normal blind 2.4
sketch "Sketch_3" plane through (0, 0, 0) normal (0, 0, 1) x (1, 0, 0)
  line L0 (-9.45, 42.9) -> (-9.45, 39.3)
  line L1 (-9.45, 39.3) -> (-9.05, 39.3)
  line L2 (-9.05, 39.3) -> (-9.05, 42.9)
  line L3 (-9.05, 42.9) -> (-9.45, 42.9)
  constraints: 8 end point
extrude "Extrusion25" add sketch "Sketch_3" against normal blind 2.4
ref_plane "1_10_XY" through (-17.9, 50.4, 2.65) normal (0, 1, 0) x (1, 0, 0)
ref_plane "1_10_YZ" through (-17.9, 50.4, 2.65) normal (1, 0, 0) x (0, 0, -1)
ref_plane "1_10_ZX" through (-17.9, 50.4, 2.65) normal (0, 0, -1) x (0, 1, 0)
ref_plane "1_11_XY" through (-17.9, 50.4, 7.65) normal (0, 1, 0) x (1, 0, 0)
ref_plane "1_11_YZ" through (-17.9, 50.4, 7.65) normal (1, 0, 0) x (0, 0, -1)
ref_plane "1_11_ZX" through (-17.9, 50.4, 7.65) normal (0, 0, -1) x (0, 1, 0)
ref_plane "1_12_XY" through (0.5, 52.4, 2.65) normal (0, 1, 0) x (1, 0, 0)
ref_plane "1_12_YZ" through (0.5, 52.4, 2.65) normal (1, 0, 0) x (0, 0, -1)
ref_plane "1_12_ZX" through (0.5, 52.4, 2.65) normal (0, 0, -1) x (0, 1, 0)
ref_plane "1_13_XY" through (0.5, 52.4, 7.65) normal (0, 1, 0) x (1, 0, 0)
ref_plane "1_13_YZ" through (0.5, 52.4, 7.65) normal (1, 0, 0) x (0, 0, -1)
ref_plane "1_13_ZX" through (0.5, 52.4, 7.65) normal (0, 0, -1) x (0, 1, 0)
ref_plane "1_14_XY" through (18.9, 54.4, 2.65) normal (0, 1, 0) x (1, 0, 0)
ref_plane "1_14_YZ" through (18.9, 54.4, 2.65) normal (1, 0, 0) x (0, 0, -1)
ref_plane "1_14_ZX" through (18.9, 54.4, 2.65) normal (0, 0, -1) x (0, 1, 0)
ref_plane "1_15_XY" through (18.9, 54.4, 7.65) normal (0, 1, 0) x (1, 0, 0)
ref_plane "1_15_YZ" through (18.9, 54.4, 7.65) normal (1, 0, 0) x (0, 0, -1)
ref_plane "1_15_ZX" through (18.9, 54.4, 7.65) normal (0, 0, -1) x (0, 1, 0)
ref_plane "1_16_XY" through (34.9, 56.4, 2.65) normal (0, 1, 0) x (1, 0, 0)
ref_plane "1_16_YZ" through (34.9, 56.4, 2.65) normal (1, 0, 0) x (0, 0, -1)
ref_plane "1_16_ZX" through (34.9, 56.4, 2.65) normal (0, 0, -1) x (0, 1, 0)
ref_plane "1_17_XY" through (34.9, 56.4, 7.65) normal (0, 1, 0) x (1, 0, 0)
ref_plane "1_17_YZ" through (34.9, 56.4, 7.65) normal (1, 0, 0) x (0, 0, -1)
ref_plane "1_17_ZX" through (34.9, 56.4, 7.65) normal (0, 0, -1) x (0, 1, 0)
ref_plane "1_18_XY" through (-12.6736, 49.904, 2.5) normal (-0.3907311, 0.9205049, 0) x (0.9205049, 0.3907311, 0)
ref_plane "1_18_YZ" through (-12.6736, 49.904, 2.5) normal (0.9205049, 0.3907311, 0) x (0, 0, -1)
ref_plane "1_18_ZX" through (-12.6736, 49.904, 2.5) normal (0, 0, -1) x (-0.3907311, 0.9205049, 0)
ref_plane "1_19_XY" through (-12.6736, 49.904, 7.5) normal (-0.3907311, 0.9205049, 0) x (0.9205049, 0.3907311, 0)
ref_plane "1_19_YZ" through (-12.6736, 49.904, 7.5) normal (0.9205049, 0.3907311, 0) x (0, 0, -1)
ref_plane "1_19_ZX" through (-12.6736, 49.904, 7.5) normal (0, 0, -1) x (-0.3907311, 0.9205049, 0)
ref_plane "1_2_XY" through (-23.7, 50.4, 2.5) normal (0, 1, 0) x (1, 0, 0)
ref_plane "1_2_YZ" through (-23.7, 50.4, 2.5) normal (1, 0, 0) x (0, 0, -1)
ref_plane "1_2_ZX" through (-23.7, 50.4, 2.5) normal (0, 0, -1) x (0, 1, 0)
ref_plane "1_20_XY" through (5.7264, 51.904, 2.5) normal (-0.3907311, 0.9205049, 0) x (0.9205049, 0.3907311, 0)
ref_plane "1_20_YZ" through (5.7264, 51.904, 2.5) normal (0.9205049, 0.3907311, 0) x (0, 0, -1)
ref_plane "1_20_ZX" through (5.7264, 51.904, 2.5) normal (0, 0, -1) x (-0.3907311, 0.9205049, 0)
ref_plane "1_21_XY" through (5.7264, 51.904, 7.5) normal (-0.3907311, 0.9205049, 0) x (0.9205049, 0.3907311, 0)
ref_plane "1_21_YZ" through (5.7264, 51.904, 7.5) normal (0.9205049, 0.3907311, 0) x (0, 0, -1)
ref_plane "1_21_ZX" through (5.7264, 51.904, 7.5) normal (0, 0, -1) x (-0.3907311, 0.9205049, 0)
ref_plane "1_22_XY" through (24.1264, 53.904, 2.5) normal (-0.3907311, 0.9205049, 0) x (0.9205049, 0.3907311, 0)
ref_plane "1_22_YZ" through (24.1264, 53.904, 2.5) normal (0.9205049, 0.3907311, 0) x (0, 0, -1)
ref_plane "1_22_ZX" through (24.1264, 53.904, 2.5) normal (0, 0, -1) x (-0.3907311, 0.9205049, 0)
ref_plane "1_23_XY" through (24.1264, 53.904, 7.5) normal (-0.3907311, 0.9205049, 0) x (0.9205049, 0.3907311, 0)
ref_plane "1_23_YZ" through (24.1264, 53.904, 7.5) normal (0.9205049, 0.3907311, 0) x (0, 0, -1)
ref_plane "1_23_ZX" through (24.1264, 53.904, 7.5) normal (0, 0, -1) x (-0.3907311, 0.9205049, 0)
ref_plane "1_24_XY" through (40.1264, 55.904, 2.5) normal (-0.3907311, 0.9205049, 0) x (0.9205049, 0.3907311, 0)
ref_plane "1_24_YZ" through (40.1264, 55.904, 2.5) normal (0.9205049, 0.3907311, 0) x (0, 0, -1)
ref_plane "1_24_ZX" through (40.1264, 55.904, 2.5) normal (0, 0, -1) x (-0.3907311, 0.9205049, 0)
ref_plane "1_25_XY" through (40.1264, 55.904, 7.5) normal (-0.3907311, 0.9205049, 0) x (0.9205049, 0.3907311, 0)
ref_plane "1_25_YZ" through (40.1264, 55.904, 7.5) normal (0.9205049, 0.3907311, 0) x (0, 0, -1)
ref_plane "1_25_ZX" through (40.1264, 55.904, 7.5) normal (0, 0, -1) x (-0.3907311, 0.9205049, 0)
ref_plane "1_28_XY" through (55.7, 60.8, 3) normal (0, 1, 0) x (1, 0, 0)
ref_plane "1_28_YZ" through (55.7, 60.8, 3) normal (1, 0, 0) x (0, 0, -1)
ref_plane "1_28_ZX" through (55.7, 60.8, 3) normal (0, 0, -1) x (0, 1, 0)
ref_plane "1_29_XY" through (55.7, 60.8, 9) normal (0, 1, 0) x (1, 0, 0)
ref_plane "1_29_YZ" through (55.7, 60.8, 9) normal (1, 0, 0) x (0, 0, -1)
ref_plane "1_29_ZX" through (55.7, 60.8, 9) normal (0, 0, -1) x (0, 1, 0)
ref_plane "1_3_XY" through (-23.7, 50.4, 7.5) normal (0, 1, 0) x (1, 0, 0)
ref_plane "1_3_YZ" through (-23.7, 50.4, 7.5) normal (1, 0, 0) x (0, 0, -1)
ref_plane "1_3_ZX" through (-23.7, 50.4, 7.5) normal (0, 0, -1) x (0, 1, 0)
ref_plane "1_4_XY" through (-5.3, 52.4, 2.5) normal (0, 1, 0) x (1, 0, 0)
ref_plane "1_4_YZ" through (-5.3, 52.4, 2.5) normal (1, 0, 0) x (0, 0, -1)
ref_plane "1_4_ZX" through (-5.3, 52.4, 2.5) normal (0, 0, -1) x (0, 1, 0)
ref_plane "1_5_XY" through (-5.3, 52.4, 7.5) normal (0, 1, 0) x (1, 0, 0)
ref_plane "1_5_YZ" through (-5.3, 52.4, 7.5) normal (1, 0, 0) x (0, 0, -1)
ref_plane "1_5_ZX" through (-5.3, 52.4, 7.5) normal (0, 0, -1) x (0, 1, 0)
ref_plane "1_6_XY" through (13.1, 54.4, 2.5) normal (0, 1, 0) x (1, 0, 0)
ref_plane "1_6_YZ" through (13.1, 54.4, 2.5) normal (1, 0, 0) x (0, 0, -1)
ref_plane "1_6_ZX" through (13.1, 54.4, 2.5) normal (0, 0, -1) x (0, 1, 0)
ref_plane "1_7_XY" through (13.1, 54.4, 7.5) normal (0, 1, 0) x (1, 0, 0)
ref_plane "1_7_YZ" through (13.1, 54.4, 7.5) normal (1, 0, 0) x (0, 0, -1)
ref_plane "1_7_ZX" through (13.1, 54.4, 7.5) normal (0, 0, -1) x (0, 1, 0)
ref_plane "1_8_XY" through (29.1, 56.4, 2.5) normal (0, 1, 0) x (1, 0, 0)
ref_plane "1_8_YZ" through (29.1, 56.4, 2.5) normal (1, 0, 0) x (0, 0, -1)
ref_plane "1_8_ZX" through (29.1, 56.4, 2.5) normal (0, 0, -1) x (0, 1, 0)
ref_plane "1_9_XY" through (29.1, 56.4, 7.5) normal (0, 1, 0) x (1, 0, 0)
ref_plane "1_9_YZ" through (29.1, 56.4, 7.5) normal (1, 0, 0) x (0, 0, -1)
ref_plane "1_9_ZX" through (29.1, 56.4, 7.5) normal (0, 0, -1) x (0, 1, 0)
sketch "Sketch38" plane through (29.1, 54.4, 2.5) normal (0, 1, 0) x (1, 0, 0)
  arc A0 (1.8119, 1.0616) -> (1.8119, -1.0616) centre (0, 0) ccw projected
sketch "Sketch39" plane through (29.1, 54.4, 7.5) normal (0, 1, 0) x (1, 0, 0)
  arc A0 (1.8119, 1.0616) -> (1.8119, -1.0616) centre (0, 0) ccw projected
sketch "Sketch40" plane through (13.1, 52.4, 2.5) normal (0, 1, 0) x (1, 0, 0)
  arc A0 (1.8119, 1.0616) -> (1.8119, -1.0616) centre (0, 0) ccw projected
sketch "Sketch41" plane through (13.1, 52.4, 7.5) normal (0, 1, 0) x (1, 0, 0)
  arc A0 (1.8119, 1.0616) -> (1.8119, -1.0616) centre (0, 0) ccw projected
sketch "Sketch42" plane through (-5.3, 50.4, 2.5) normal (0, 1, 0) x (1, 0, 0)
  arc A0 (1.8119, 1.0616) -> (1.8119, -1.0616) centre (0, 0) ccw projected
sketch "Sketch43" plane through (-5.3, 50.4, 7.5) normal (0, 1, 0) x (1, 0, 0)
  arc A0 (1.8119, 1.0616) -> (1.8119, -1.0616) centre (0, 0) ccw projected
sketch "Sketch44" plane through (-23.7, 48.4, 2.5) normal (0, 1, 0) x (1, 0, 0)
  arc A0 (1.8119, 1.0616) -> (1.8119, -1.0616) centre (0, 0) ccw projected
sketch "Sketch45" plane through (-23.7, 48.4, 7.5) normal (0, 1, 0) x (1, 0, 0)
  arc A0 (1.8119, 1.0616) -> (1.8119, -1.0616) centre (0, 0) ccw projected
body "Solid1"
